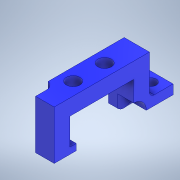
# Autodesk Inventor part: Servo mount
Saved by Autodesk Inventor 2022.6 (Build 266554000, 554)
## iProperties
Created: 2024-11-05
Part Number: Servo mount
Material: Generic
Document SubType Name: Modeling
Designer: Admin
Density: 1 g/cm^3
Appearance: Blue - Wall Paint - Glossy
Author: Admin
Autodesk Inventor part; units mm, degrees
ref_plane "YZ Plane" through (0, 0, 0) normal (1, 0, 0) x (0, 1, 0)
ref_plane "XZ Plane" through (0, 0, 0) normal (0, 1, 0) x (-1, 0, 0)
ref_plane "XY Plane" through (0, 0, 0) normal (0, 0, 1) x (1, 0, 0)
sketch "Sketch1" plane through (0, 0, 0) normal (1, 0, 0) x (0, 1, 0)
  line L0 (0, 0) -> (15.5, 0)
  line L1 (15.5, 0) -> (15.5, -5)
  line L2 (15.5, -5) -> (0, -5)
  line L3 (0, -5) -> (0, 0)
  line L4 (15.5, 0) -> (10.5, 0)
  line L5 (10.5, 0) -> (10.5, 20.2)
  line L6 (10.5, 20.2) -> (15.5, 20.2)
  line L7 (15.5, 20.2) -> (15.5, 0)
  line L8 (15.5, 20.2) -> (0, 20.2)
  line L9 (0, 20.2) -> (0, 25.2)
  line L10 (0, 25.2) -> (15.5, 25.2)
  line L11 (15.5, 25.2) -> (15.5, 20.2)
  line L12 (2, 20.2) -> (0, 20.2)
  line L13 (0, 20.2) -> (0, 18.2)
  line L14 (0, 18.2) -> (2, 18.2)
  line L15 (2, 18.2) -> (2, 20.2)
  dimension "d0" = 5
  dimension "d2" = 5
  dimension "d3" = 20.2
  dimension "d4" = 5
  dimension "d16" = 10.5
  dimension "d23" = 2
  dimension "d24" = 2
  constraints: 32 end point, 9 parallel, 4 horizontal, 4 perpendicular, 1 point on line
  measures "d0" distance of L0.end L1.end
  measures "d2" distance of L5.end L6.end
  measures "d3" distance of L6.end L0.end
  measures "d4" distance of L8.end L9.end
  measures "d16" distance between parallel lines of L3 L5
  measures "d23" distance of L14.end L13.end
  measures "d24" distance of L14.end L12.start
extrude "Extrusion1" add sketch "Sketch1" along normal blind 8
sketch "Sketch2" plane through (0, 15.5, 25.2) normal (0, 1, 0) x (1, 0, 0)
  line L0 (0, 0) -> (8, 0) construction
  line L1 (3.9, 0) -> (3.9, 30.2) construction
  line L2 (0, 30.2) -> (8, 30.2) construction
  line L3 (0, 30.2) -> (0, 0) construction
  line L4 (0, 30.2) -> (0, 0) construction
  line L5 (0, 0) -> (8, 0) construction
  line L6 (8, 30.2) -> (8, 0) construction
  line L7 (0, 30.2) -> (8, 30.2) construction
  line L8 (3.9, 15.1) -> (1.5202, 15.1)
  point P0 (0, 25.2)
  point P1 (3.9, 10.1)
  point P2 (3.9, 20.1)
  dimension "d7" = 3.9
  dimension "d8" = 10
  constraints: 4 end point, 4 point on line, 1 horizontal, 1 midpoint, 1 symmetric about line, 1 vertical
  measures "d7" distance between parallel lines of L3 L1
  measures "d8" distance of point (3.9, 10.1) point (3.9, 20.1)
hole "Hole1" at (3.9, 15.5, 15.1) at (3.9, 15.5, 5.1) direction (0, -1, 0) diameter 4.3 depth 10 tip angle 118
sketch "Sketch4" plane through (0, 15.5, 25.2) normal (0, 1, 0) x (1, 0, 0)
  circle A0 centre (3.9, 10.1) radius 2.15 projected
  circle A1 centre (3.9, 20.1) radius 2.15 projected
  line L0 (0, 30.2) -> (0, 0) projected
  line L1 (0, 0) -> (8, 0) projected
  line L2 (8, 30.2) -> (8, 0) projected
  line L3 (0, 30.2) -> (8, 30.2) projected
  line L4 (0, 0) -> (8, 0) projected
  circle A2 centre (-0.5, 3.5) radius 2.6
  line L5 (2.1, 3.5) -> (2.1, 0)
  point P0 (0, 25.2)
  point P1 (0, 6.0515)
  point P2 (0, 0.9485)
  point P3 (2.1, 0)
  dimension "d19" = 5.2
  dimension "d20" = 0.5
  dimension "d63" = 3.5
  constraints: 2 end point, 1 perpendicular, 1 point on line, 1 vertical, 3 other
  measures "d20" distance from line of L0 point (-0.5, 3.5)
  measures "d63" distance from line of L1 point (-0.5, 3.5)
extrude "Extrusion2" cut sketch "Sketch4" against normal through all contours A2 L0 | A2 L5 L1 L0 picked at (0.1891, 2.7097)
sketch "Sketch5" plane through (0, 0, 18.2) normal (0, -1, 0) x (1, 0, 0)
  arc A0 (0, 0.9485) -> (2.1, 3.5) centre (-0.5, 3.5) ccw projected
  line L0 (0, 0.9485) -> (0, 0) projected
  line L1 (0, 0) -> (8, 0) projected
  line L2 (8, 7) -> (8, 0) projected
  line L3 (2.1, 7) -> (8, 7) projected
  line L4 (2.1, 7) -> (2.1, 3.5) projected
  circle A1 centre (4, 4) radius 1.4
  point P0 (0, -18.2)
  point P1 (8, 3.5)
  dimension "d25" = 2.8
  dimension "d26" = 4
  dimension "d28" = 3
  constraints: 1 centre point, 1 midpoint
  measures "d25" diameter of A1
  measures "d26" horizontal distance of point (8, 3.5) A1.centre
  measures "d28" distance from line of L3 A1.centre
extrude "Extrusion3" add sketch "Sketch5" along normal blind 1.5 contours A1
sketch "Sketch6" plane through (0, 0, -5) normal (0, -1, 0) x (1, 0, 0)
  line L0 (0, 5) -> (0, 0) projected
  line L1 (0, 0) -> (8, 0) projected
  line L2 (8, 5) -> (8, 0) projected
  line L3 (0, 5) -> (8, 5) projected
  line L4 (0, 5) -> (8, 5) projected
  line L5 (0, 0) -> (0, 24.1485) projected
  line L6 (8, 0) -> (-7, 0)
  line L7 (-7, 0) -> (-7, -7.5)
  line L8 (-7, -7.5) -> (8, -7.5)
  line L9 (8, -7.5) -> (8, 0)
  dimension "d59" = 7.5
  dimension "d60" = 15
  constraints: 8 end point, 2 parallel, 1 horizontal, 1 perpendicular
  measures "d59" distance of L7.end L6.end
  measures "d60" distance of L7.end L8.end
extrude "Extrusion4" add sketch "Sketch6" against normal blind 3 contours L1 L9 L8 L7 L6
fillet "Fillet1" radius 1.5 2 edges at (4, 3, -5) (0, 1.5, -5)
sketch "Sketch9" plane through (8, 0, 0) normal (1, 0, 0) x (0, 0, -1)
  line L0 (0, 0) -> (3.5, 0) projected
  circle A0 centre (0, 0) radius 4
  dimension "d64" = 8
  constraints: 1 centre point, 1 coincident
  measures "d64" diameter of A0
extrude "Extrusion5" cut sketch "Sketch9" against normal blind 3
fillet "Fillet2" radius 2 2 edges at (5, 0, -2) (5, 2, 0)
sketch "Sketch10" plane through (-7, 0, -12.5) normal (0, -1, 0) x (1, 0, 0)
  line L0 (10, 12.5) -> (10, 8.5) projected
  line L1 (7, 12.5) -> (10, 12.5) projected
  line L2 (7, 12.5) -> (7, 9) projected
  arc A0 (5.5, 7.5) -> (7, 9) centre (5.5, 9) ccw projected
  line L3 (5.5, 7.5) -> (0, 7.5) projected
  line L4 (0, 7.5) -> (0, 0) projected
  line L5 (0, 0) -> (15, 0) projected
  line L6 (15, 8.5) -> (15, 0) projected
  line L7 (15, 8.5) -> (10, 8.5) projected
  line L8 (15, 0) -> (0, 0) construction
  line L9 (0, 7.5) -> (5.5, 7.5) construction
  point P0 (11, 3)
  point P1 (2.75, 3)
  dimension "d76" = 3
  dimension "d77" = 4
  constraints: 1 horizontal alignment
  measures "d76" distance from line of L5 point (2.75, 3)
  measures "d77" distance from line of L6 point (11, 3)
hole "Hole4" at (4, 0, -9.5) at (-4.25, 0, -9.5) direction (0, 1, 0) diameter 3.4 depth 10 tip angle 118
body "Solid1"
